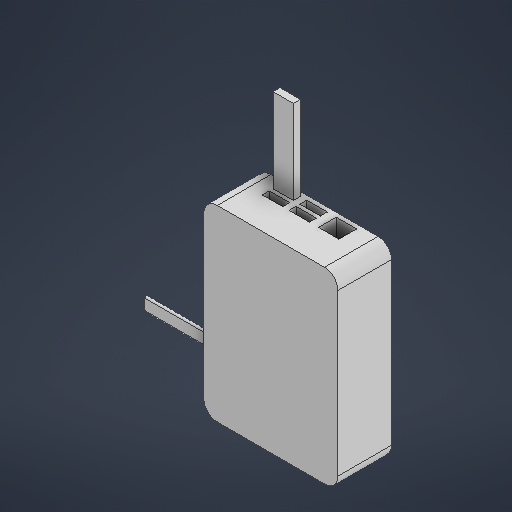
# Autodesk Inventor part: RaspberryPi
Saved by Autodesk Inventor 2026.2 (Build 302298000, 298)
## iProperties
Created: 2026-01-21
Part Number: RaspberryPi
Material: Generic
Document SubType Name: Modeling
Designer: User
Density: 1 g/cm^3
Appearance: Default
Author: User
Autodesk Inventor part; units mm, degrees
ref_plane "YZ Plane" through (0, 0, 0) normal (1, 0, 0) x (0, 1, 0)
ref_plane "XZ Plane" through (0, 0, 0) normal (0, 1, 0) x (-1, 0, 0)
ref_plane "XY Plane" through (0, 0, 0) normal (0, 0, 1) x (1, 0, 0)
sketch "Sketch1" plane through (0, 0, 0) normal (0, 0, 1) x (1, 0, 0)
  line L0 (6.35, 0) -> (57.15, 0)
  line L1 (63.5, 6.35) -> (63.5, 82.55)
  line L2 (57.15, 88.9) -> (6.35, 88.9)
  line L3 (0, 82.55) -> (0, 6.35)
  arc A0 (6.35, 88.9) -> (0, 82.55) centre (6.35, 82.55) ccw
  arc A1 (63.5, 82.55) -> (57.15, 88.9) centre (57.15, 82.55) ccw
  arc A2 (57.15, 0) -> (63.5, 6.35) centre (57.15, 6.35) ccw
  arc A3 (0, 6.35) -> (6.35, 0) centre (6.35, 6.35) ccw
  point P0 (0, 0)
  point P1 (63.5, 88.9)
  point P2 (63.5, 0)
  point P3 (0, 88.9)
  dimension "d0" = 88.9
  dimension "d1" = 63.5
  dimension "d2" = 6.35
  constraints: 8 end point, 8 point on circle, 8 point on line, 8 tangent, 4 centre point, 3 equal radius, 2 parallel, 1 horizontal, 1 perpendicular
  measures "d0" distance of point (63.5, 0) point (63.5, 88.9)
  measures "d1" distance of point (63.5, 88.9) point (0, 88.9)
  measures "d2" radius of A0
extrude "Extrusion1" add sketch "Sketch1" along normal blind 25.4
sketch "Sketch2" plane through (6.35, 88.9, 0) normal (0, 1, 0) x (1, 0, 0)
  line L0 (6.35, -2.032) -> (16.002, -2.032)
  line L1 (16.002, -2.032) -> (16.002, -5.334)
  line L2 (16.002, -5.334) -> (6.35, -5.334)
  line L3 (6.35, -5.334) -> (6.35, -2.032)
  line L4 (0, 0) -> (0, -25.4) projected
  line L5 (50.8, 0) -> (0, 0) projected
  line L6 (28.702, -5.334) -> (19.05, -5.334)
  line L7 (19.05, -2.032) -> (28.702, -2.032)
  line L8 (28.702, -2.032) -> (28.702, -5.334)
  line L9 (19.05, -5.334) -> (19.05, -2.032)
  line L10 (16.002, -10.414) -> (6.35, -10.414)
  line L11 (6.35, -7.112) -> (16.002, -7.112)
  line L12 (16.002, -7.112) -> (16.002, -10.414)
  line L13 (6.35, -10.414) -> (6.35, -7.112)
  line L14 (28.702, -10.414) -> (19.05, -10.414)
  line L15 (19.05, -7.112) -> (28.702, -7.112)
  line L16 (28.702, -7.112) -> (28.702, -10.414)
  line L17 (19.05, -10.414) -> (19.05, -7.112)
  line L18 (33.02, -2.032) -> (42.672, -2.032)
  line L19 (42.672, -2.032) -> (42.672, -10.414)
  line L20 (42.672, -10.414) -> (33.02, -10.414)
  line L21 (33.02, -10.414) -> (33.02, -2.032)
  point P0 (-6.35, 0)
  point P1 (6.35, -3.683)
  point P2 (19.05, -3.683)
  point P3 (6.35, -8.763)
  point P4 (19.05, -8.763)
  point P5 (37.846, -2.032)
  dimension "d5" = 6.35
  dimension "d6" = 9.652
  dimension "d7" = 3.302
  dimension "d8" = 2.032
  dimension "d11" = 12.7
  dimension "d14" = 5.08
  dimension "d17" = 8.382
  dimension "d18" = 9.652
  dimension "d19" = 4.318
  dimension "d20" = 0
  constraints: 40 end point, 4 parallel, 3 horizontal, 2 midpoint, 2 perpendicular, 1 vertical, 27 other
  measures "d5" distance from line of L4 point (6.35, -3.683)
  measures "d6" distance of L0.start L0.end
  measures "d7" distance of L0.end L1.end
  measures "d8" distance between parallel lines of L5 L0
  measures "d11" distance of L1.end L6.start
  measures "d14" distance of L1.end L10.start
  measures "d17" distance of L18.end L19.end
  measures "d18" distance of L18.start L18.end
  measures "d19" distance between parallel lines of L8 L21
  measures "d20" distance from line of point (37.846, -2.032) L7
extrude "Extrusion2" cut sketch "Sketch2" against normal blind 10.16
sketch "Sketch3" plane through (0, 6.35, 0) normal (-1, 0, 0) x (0, 0, 1)
  line L0 (12.7, 10.16) -> (12.7, 15.24) construction
  line L1 (12.065, 10.16) -> (12.065, 15.24)
  line L2 (13.335, 15.24) -> (13.335, 10.16)
  arc A0 (12.065, 10.16) -> (13.335, 10.16) centre (12.7, 10.16) ccw
  arc A1 (13.335, 15.24) -> (12.065, 15.24) centre (12.7, 15.24) ccw
  line L3 (25.4, 76.2) -> (25.4, 0) projected
  line L4 (0, 0) -> (25.4, 0) projected
  line L5 (13.335, 27.94) -> (13.335, 22.86)
  arc A2 (12.065, 22.86) -> (13.335, 22.86) centre (12.7, 22.86) ccw
  line L6 (12.065, 22.86) -> (12.065, 27.94)
  arc A3 (13.335, 27.94) -> (12.065, 27.94) centre (12.7, 27.94) ccw
  line L7 (13.335, 40.64) -> (13.335, 35.56)
  arc A4 (12.065, 35.56) -> (13.335, 35.56) centre (12.7, 35.56) ccw
  line L8 (12.065, 35.56) -> (12.065, 40.64)
  arc A5 (13.335, 40.64) -> (12.065, 40.64) centre (12.7, 40.64) ccw
  circle A6 centre (12.7, 50.8) radius 2.286
  line L9 (0, 76.2) -> (25.4, 76.2) projected
  point P0 (0, -6.35)
  point P1 (12.7, 12.7)
  point P2 (12.7, 76.2)
  dimension "d23" = 5.08
  dimension "d24" = 0.635
  dimension "d25" = 12.7
  dimension "d26" = 12.7
  dimension "d29" = 12.7
  dimension "d34" = 4.572
  dimension "d35" = 12.7
  dimension "d36" = 25.4
  constraints: 16 end point, 12 point on circle, 7 centre point, 4 tangent, 2 midpoint, 2 vertical, 1 parallel, 20 other
  measures "d23" distance of L1.start L1.end
  measures "d24" radius of A1
  measures "d25" distance from line of L3 point (12.7, 12.7)
  measures "d26" distance from line of L4 point (12.7, 12.7)
  measures "d29" distance of L2.start L5.start
  measures "d34" diameter of A6
  measures "d35" distance from line of L3 A6.centre
  measures "d36" distance of point (12.7, 76.2) A6.centre
extrude "Extrusion3" cut sketch "Sketch3" against normal blind 10.16
sketch "Sketch4" plane through (6.35, 78.74, 0) normal (0, 1, 0) x (1, 0, 0)
  point P0 (-6.35, 0)
sketch "Sketch5" plane through (6.35, 78.74, 0) normal (0, 1, 0) x (1, 0, 0)
  line L0 (16.002, -5.334) -> (6.35, -5.334) projected
  line L1 (6.35, -5.334) -> (6.35, -2.032) projected
  line L2 (6.35, -2.032) -> (16.002, -2.032) projected
  line L3 (16.002, -2.032) -> (16.002, -5.334) projected
  point P0 (-6.35, 0)
extrude "Extrusion4" add sketch "Sketch5" along normal blind 50
sketch "Sketch6" plane through (0, 6.35, 0) normal (-1, 0, 0) x (0, 0, 1)
  arc A0 (12.065, 10.16) -> (13.335, 10.16) centre (12.7, 10.16) ccw projected
  line L0 (13.335, 15.24) -> (13.335, 10.16) projected
  line L1 (12.065, 10.16) -> (12.065, 15.24) projected
  arc A1 (13.335, 15.24) -> (12.065, 15.24) centre (12.7, 15.24) ccw projected
  arc A2 (12.065, 22.86) -> (13.335, 22.86) centre (12.7, 22.86) ccw projected
  line L2 (13.335, 27.94) -> (13.335, 22.86) projected
  line L3 (12.065, 22.86) -> (12.065, 27.94) projected
  arc A3 (13.335, 27.94) -> (12.065, 27.94) centre (12.7, 27.94) ccw projected
  point P0 (0, -6.35)
extrude "Extrusion5" add sketch "Sketch6" along normal blind 40 contours L1 A1 L0 A0
sketch "Sketch7" plane through (0, 0, 0) normal (0, 0, -1) x (-1, 0, 0)
  line L0 (-54.5456, 57.3368) -> (-7.6923, 57.3368) construction
  line L1 (-7.6923, 57.3368) -> (-7.6923, 33.9102) construction
  line L2 (-7.6923, 33.9102) -> (-54.5456, 33.9102) construction
  line L3 (-54.5456, 33.9102) -> (-54.5456, 57.3368) construction
  line L4 (-53.5254, 54.2246) -> (-53.5254, 56.912)
  line L5 (-53.5254, 56.912) -> (-54.548, 56.912)
  line L6 (-54.548, 56.912) -> (-54.548, 57.2726)
  line L7 (-54.548, 57.2726) -> (-52.0978, 57.2726)
  line L8 (-52.0978, 57.2726) -> (-52.0978, 56.912)
  line L9 (-52.0978, 56.912) -> (-53.1204, 56.912)
  line L10 (-53.1204, 56.912) -> (-53.1204, 54.2246)
  line L11 (-53.1204, 54.2246) -> (-53.5254, 54.2246)
  spline S0 degree 2 poles (-49.6327, 56.9243) (-49.4598, 56.7218) (-49.2671, 56.129) (-49.2671, 55.7486) knots 0 0 0 1 2 2 2
  spline S1 degree 2 poles (-49.2671, 55.7486) (-49.2671, 55.3781) (-49.4549, 54.7779) (-49.6327, 54.5753) knots 0 0 0 1 2 2 2
  spline S2 degree 2 poles (-49.6327, 54.5753) (-49.8204, 54.3629) (-50.3169, 54.1604) (-50.6158, 54.1604) knots 0 0 0 1 2 2 2
  spline S3 degree 2 poles (-50.6158, 54.1604) (-50.9245, 54.1604) (-51.4185, 54.3703) (-51.5988, 54.5753) knots 0 0 0 1 2 2 2
  spline S4 degree 2 poles (-51.5988, 54.5753) (-51.7742, 54.7779) (-51.9619, 55.3731) (-51.9619, 55.7486) knots 0 0 0 1 2 2 2
  spline S5 degree 2 poles (-51.9619, 55.7486) (-51.9619, 56.1314) (-51.7717, 56.7144) (-51.5964, 56.9243) knots 0 0 0 1 2 2 2
  spline S6 degree 2 poles (-51.5964, 56.9243) (-51.4185, 57.1269) (-50.9221, 57.3368) (-50.6158, 57.3368) knots 0 0 0 1 2 2 2
  spline S7 degree 2 poles (-50.6158, 57.3368) (-50.3045, 57.3368) (-49.8056, 57.1194) (-49.6327, 56.9243) knots 0 0 0 1 2 2 2
  spline S8 degree 2 poles (-49.6895, 55.7486) (-49.6895, 56.0499) (-49.8204, 56.5168) (-49.939, 56.6699) knots 0 0 0 1 2 2 2
  spline S9 degree 2 poles (-49.939, 56.6699) (-50.06, 56.828) (-50.4009, 56.9861) (-50.6133, 56.9861) knots 0 0 0 1 2 2 2
  spline S10 degree 2 poles (-50.6133, 56.9861) (-50.8331, 56.9861) (-51.1641, 56.8329) (-51.2901, 56.6699) knots 0 0 0 1 2 2 2
  spline S11 degree 2 poles (-51.2901, 56.6699) (-51.4111, 56.5143) (-51.5396, 56.045) (-51.5396, 55.7486) knots 0 0 0 1 2 2 2
  spline S12 degree 2 poles (-51.5396, 55.7486) (-51.5396, 55.1484) (-51.0357, 54.5111) (-50.6133, 54.5111) knots 0 0 0 1 2 2 2
  spline S13 degree 2 poles (-50.6133, 54.5111) (-50.1909, 54.5111) (-49.6895, 55.1484) (-49.6895, 55.7486) knots 0 0 0 1 2 2 2
  spline S14 degree 2 poles (-46.8959, 56.3537) (-46.8959, 56.1561) (-47.0367, 55.8005) (-47.1627, 55.677) knots 0 0 0 1 2 2 2
  spline S15 degree 2 poles (-47.1627, 55.677) (-47.3208, 55.5213) (-47.7481, 55.3608) (-48.0741, 55.3608) knots 0 0 0 1 2 2 2
  line L12 (-48.0741, 55.3608) -> (-48.4175, 55.3608)
  line L13 (-48.4175, 55.3608) -> (-48.4175, 54.2246)
  line L14 (-48.4175, 54.2246) -> (-48.8225, 54.2246)
  line L15 (-48.8225, 54.2246) -> (-48.8225, 57.2726)
  line L16 (-48.8225, 57.2726) -> (-48.0568, 57.2726)
  spline S16 degree 2 poles (-48.0568, 57.2726) (-47.7851, 57.2726) (-47.4047, 57.1837) (-47.259, 57.0824) knots 0 0 0 1 2 2 2
  spline S17 degree 2 poles (-47.259, 57.0824) (-47.0886, 56.9663) (-46.8959, 56.6082) (-46.8959, 56.3537) knots 0 0 0 1 2 2 2
  spline S18 degree 2 poles (-47.3183, 56.3414) (-47.3183, 56.4995) (-47.427, 56.7317) (-47.5381, 56.8058) knots 0 0 0 1 2 2 2
  spline S19 degree 2 poles (-47.5381, 56.8058) (-47.6345, 56.87) (-47.8913, 56.9218) (-48.0815, 56.9218) knots 0 0 0 1 2 2 2
  line L17 (-48.0815, 56.9218) -> (-48.4175, 56.9218)
  line L18 (-48.4175, 56.9218) -> (-48.4175, 55.7066)
  line L19 (-48.4175, 55.7066) -> (-48.1408, 55.7066)
  spline S20 degree 2 poles (-48.1408, 55.7066) (-47.8938, 55.7066) (-47.59, 55.7856) (-47.4912, 55.8894) knots 0 0 0 1 2 2 2
  spline S21 degree 2 poles (-47.4912, 55.8894) (-47.3998, 55.9808) (-47.3183, 56.1957) (-47.3183, 56.3414) knots 0 0 0 1 2 2 2
  point P0 (0, 0)
  dimension "d0" = 88.9
  dimension "d1" = 63.5
  dimension "d2" = 6.35
  constraints: 2 other
extrude "Extrusion6" add sketch "Sketch7" along normal blind 0.5
body "Solid1"
